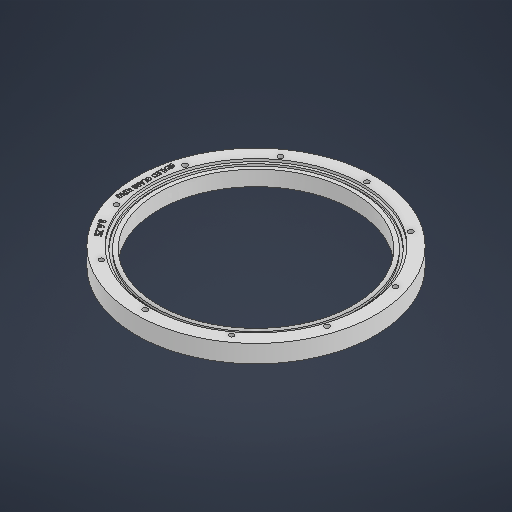
# Autodesk Inventor part: SealedGlassRing
Saved by Autodesk Inventor 2026.1 (Build 301233000, 233)
## iProperties
Created: 2025-06-19
Part Number: SealedGlassRing
Material: Generic
Document SubType Name: Modeling
Designer: mumin
Density: 1 g/cm^3
Appearance: Default
Author: mumin
Autodesk Inventor part; units mm, degrees
ref_plane "YZ Plane" through (0, 0, 0) normal (1, 0, 0) x (0, 1, 0)
ref_plane "XZ Plane" through (0, 0, 0) normal (0, 1, 0) x (-1, 0, 0)
ref_plane "XY Plane" through (0, 0, 0) normal (0, 0, 1) x (1, 0, 0)
sketch "Sketch1" plane through (0, 0, 0) normal (0, 1, 0) x (-1, 0, 0)
  circle A0 centre (0, 0) radius 110
  circle A1 centre (0, 0) radius 135
  dimension "d0" = 220
  dimension "d1" = 270
  constraints: 2 centre point, 2 coincident
  measures "d0" diameter of A0
  measures "d1" diameter of A1
extrude "Ring" add sketch "Sketch1" along normal blind 20
sketch "Sketch2" plane through (0, 20, 0) normal (0, 1, 0) x (1, 0, 0)
  circle A0 centre (0, 0) radius 120.5
  dimension "d4" = 241
  constraints: 1 centre point, 1 coincident
  measures "d4" diameter of A0
extrude "Glass Seat" cut sketch "Sketch2" against normal blind 2.95
sketch "Sketch3" plane through (0, 20, 0) normal (0, 1, 0) x (1, 0, 0)
  line L0 (0, 189) -> (0, -189) projected
  point P0 (0, 0)
  point P1 (0, 125)
  dimension "d14" = 125
  constraints: 1 point on line
  measures "d14" distance of point (0, 0) point (0, 125)
hole "Holes" at (0, 20, -125) direction (0, -1, 0) diameter 5.5 end through all
pattern_circular "Circular Pattern1" count 10 over 360 about axis through (0, -10, 0) along (0, 1, 0) of "Holes"
sketch "Sketch4" plane through (0, 20, 0) normal (0, 1, 0) x (1, 0, 0)
  line L0 (-123.4008, 33.078) -> (-123.4008, -40.8071) construction
  line L1 (-123.4008, -40.8071) -> (-126.5772, -40.8071) construction
  line L2 (-126.5772, -40.8071) -> (-126.5772, 33.078) construction
  line L3 (-126.5772, 33.078) -> (-123.4008, 33.078) construction
  spline S0 degree 2 poles (-128.5791, 31.1777) (-128.5791, 31.7207) (-128.3522, 32.4824) (-128.1901, 32.8187) knots 0 0 0 1 2 2 2
  line L4 (-128.1901, 32.8187) -> (-127.3554, 32.8187)
  line L5 (-127.3554, 32.8187) -> (-127.3554, 32.7701)
  spline S1 degree 2 poles (-127.3554, 32.7701) (-127.6634, 32.4419) (-128.0037, 31.6113) (-128.0037, 31.2263) knots 0 0 0 1 2 2 2
  spline S2 degree 2 poles (-128.0037, 31.2263) (-128.0037, 30.6753) (-127.5459, 30.1121) (-127.169, 30.1121) knots 0 0 0 1 2 2 2
  spline S3 degree 2 poles (-127.169, 30.1121) (-126.8692, 30.1121) (-126.4964, 30.4079) (-126.4032, 30.7279) knots 0 0 0 1 2 2 2
  spline S4 degree 2 poles (-126.4032, 30.7279) (-126.3384, 30.9589) (-126.2493, 31.3438) (-126.1763, 31.6315) knots 0 0 0 1 2 2 2
  spline S5 degree 2 poles (-126.1763, 31.6315) (-126.1074, 31.8908) (-125.9008, 32.3001) (-125.7347, 32.4581) knots 0 0 0 1 2 2 2
  spline S6 degree 2 poles (-125.7347, 32.4581) (-125.5685, 32.6121) (-125.1228, 32.7822) (-124.8311, 32.7822) knots 0 0 0 1 2 2 2
  spline S7 degree 2 poles (-124.8311, 32.7822) (-124.2233, 32.7822) (-123.4008, 31.8341) (-123.4008, 31.1007) knots 0 0 0 1 2 2 2
  spline S8 degree 2 poles (-123.4008, 31.1007) (-123.4008, 30.6793) (-123.5669, 29.9338) (-123.7249, 29.6137) knots 0 0 0 1 2 2 2
  line L6 (-123.7249, 29.6137) -> (-124.5191, 29.6137)
  line L7 (-124.5191, 29.6137) -> (-124.5191, 29.6623)
  spline S9 degree 2 poles (-124.5191, 29.6623) (-124.3003, 29.9014) (-123.9762, 30.6469) (-123.9762, 31.0561) knots 0 0 0 1 2 2 2
  spline S10 degree 2 poles (-123.9762, 31.0561) (-123.9762, 31.5181) (-124.4097, 32.0894) (-124.7622, 32.0894) knots 0 0 0 1 2 2 2
  spline S11 degree 2 poles (-124.7622, 32.0894) (-125.0783, 32.0894) (-125.4551, 31.7531) (-125.5402, 31.437) knots 0 0 0 1 2 2 2
  spline S12 degree 2 poles (-125.5402, 31.437) (-125.5969, 31.2263) (-125.7428, 30.6145) (-125.8036, 30.4119) knots 0 0 0 1 2 2 2
  spline S13 degree 2 poles (-125.8036, 30.4119) (-125.9616, 29.8973) (-126.5977, 29.4192) (-127.0637, 29.4192) knots 0 0 0 1 2 2 2
  spline S14 degree 2 poles (-127.0637, 29.4192) (-127.3595, 29.4192) (-127.9267, 29.6583) (-128.1253, 29.873) knots 0 0 0 1 2 2 2
  spline S15 degree 2 poles (-128.1253, 29.873) (-128.3441, 30.1121) (-128.5791, 30.7198) (-128.5791, 31.1777) knots 0 0 0 1 2 2 2
  line L8 (-128.4899, 28.7425) -> (-123.4899, 28.7425)
  line L9 (-123.4899, 28.7425) -> (-123.4899, 25.6145)
  line L10 (-123.4899, 25.6145) -> (-124.0815, 25.6145)
  line L11 (-124.0815, 25.6145) -> (-124.0815, 28.078)
  line L12 (-124.0815, 28.078) -> (-125.451, 28.078)
  line L13 (-125.451, 28.078) -> (-125.451, 25.7806)
  line L14 (-125.451, 25.7806) -> (-126.0426, 25.7806)
  line L15 (-126.0426, 25.7806) -> (-126.0426, 28.078)
  line L16 (-126.0426, 28.078) -> (-127.8984, 28.078)
  line L17 (-127.8984, 28.078) -> (-127.8984, 25.6145)
  line L18 (-127.8984, 25.6145) -> (-128.4899, 25.6145)
  line L19 (-128.4899, 25.6145) -> (-128.4899, 28.7425)
  line L20 (-128.4899, 25.4241) -> (-123.4899, 23.7385)
  line L21 (-123.4899, 23.7385) -> (-123.4899, 22.92)
  line L22 (-123.4899, 22.92) -> (-128.4899, 21.2344)
  line L23 (-128.4899, 21.2344) -> (-128.4899, 21.9354)
  line L24 (-128.4899, 21.9354) -> (-127.092, 22.3892)
  line L25 (-127.092, 22.3892) -> (-127.092, 24.2976)
  line L26 (-127.092, 24.2976) -> (-128.4899, 24.7514)
  line L27 (-128.4899, 24.7514) -> (-128.4899, 25.4241)
  line L28 (-126.5248, 22.5715) -> (-124.1707, 23.3455)
  line L29 (-124.1707, 23.3455) -> (-126.5248, 24.1153)
  line L30 (-126.5248, 24.1153) -> (-126.5248, 22.5715)
  line L31 (-128.4899, 17.8633) -> (-128.4899, 20.7604)
  line L32 (-128.4899, 20.7604) -> (-123.4899, 20.7604)
  line L33 (-123.4899, 20.7604) -> (-123.4899, 20.0959)
  line L34 (-123.4899, 20.0959) -> (-127.8984, 20.0959)
  line L35 (-127.8984, 20.0959) -> (-127.8984, 17.8633)
  line L36 (-127.8984, 17.8633) -> (-128.4899, 17.8633)
  line L37 (-128.4899, 17.3406) -> (-123.4899, 17.3406)
  line L38 (-123.4899, 17.3406) -> (-123.4899, 14.2126)
  line L39 (-123.4899, 14.2126) -> (-124.0815, 14.2126)
  line L40 (-124.0815, 14.2126) -> (-124.0815, 16.6761)
  line L41 (-124.0815, 16.6761) -> (-125.451, 16.6761)
  line L42 (-125.451, 16.6761) -> (-125.451, 14.3787)
  line L43 (-125.451, 14.3787) -> (-126.0426, 14.3787)
  line L44 (-126.0426, 14.3787) -> (-126.0426, 16.6761)
  line L45 (-126.0426, 16.6761) -> (-127.8984, 16.6761)
  line L46 (-127.8984, 16.6761) -> (-127.8984, 14.2126)
  line L47 (-127.8984, 14.2126) -> (-128.4899, 14.2126)
  line L48 (-128.4899, 14.2126) -> (-128.4899, 17.3406)
  spline S16 degree 2 poles (-125.994, 9.5408) (-126.6788, 9.5408) (-127.7809, 10.0959) (-128.0888, 10.5618) knots 0 0 0 1 2 2 2
  spline S17 degree 2 poles (-128.0888, 10.5618) (-128.3279, 10.9427) (-128.4899, 11.7247) (-128.4899, 12.3325) knots 0 0 0 1 2 2 2
  line L49 (-128.4899, 12.3325) -> (-128.4899, 13.4832)
  line L50 (-128.4899, 13.4832) -> (-123.4899, 13.4832)
  line L51 (-123.4899, 13.4832) -> (-123.4899, 12.3446)
  spline S18 degree 2 poles (-123.4899, 12.3446) (-123.4899, 11.6396) (-123.7006, 10.8373) (-123.887, 10.5537) knots 0 0 0 1 2 2 2
  spline S19 degree 2 poles (-123.887, 10.5537) (-124.2071, 10.0715) (-125.2647, 9.5408) (-125.994, 9.5408) knots 0 0 0 1 2 2 2
  spline S20 degree 2 poles (-125.9859, 10.2336) (-125.4105, 10.2336) (-124.5961, 10.6145) (-124.3651, 10.9913) knots 0 0 0 1 2 2 2
  spline S21 degree 2 poles (-124.3651, 10.9913) (-124.2071, 11.2587) (-124.0653, 11.8625) (-124.0653, 12.3122) knots 0 0 0 1 2 2 2
  line L52 (-124.0653, 12.3122) -> (-124.0653, 12.8187)
  line L53 (-124.0653, 12.8187) -> (-127.9146, 12.8187)
  line L54 (-127.9146, 12.8187) -> (-127.9146, 12.3122)
  spline S22 degree 2 poles (-127.9146, 12.3122) (-127.9146, 11.8706) (-127.7728, 11.202) (-127.5823, 10.9305) knots 0 0 0 1 2 2 2
  spline S23 degree 2 poles (-127.5823, 10.9305) (-127.3473, 10.5821) (-126.5694, 10.2336) (-125.9859, 10.2336) knots 0 0 0 1 2 2 2
  spline S24 degree 2 poles (-128.5872, 4.5772) (-128.5872, 5.108) (-128.263, 5.9873) (-127.9348, 6.3033) knots 0 0 0 1 2 2 2
  spline S25 degree 2 poles (-127.9348, 6.3033) (-127.6026, 6.6194) (-126.622, 6.9557) (-125.9859, 6.9557) knots 0 0 0 1 2 2 2
  spline S26 degree 2 poles (-125.9859, 6.9557) (-125.3822, 6.9557) (-124.4259, 6.6153) (-124.0856, 6.2993) knots 0 0 0 1 2 2 2
  spline S27 degree 2 poles (-124.0856, 6.2993) (-123.7574, 5.9954) (-123.4008, 5.104) (-123.4008, 4.5732) knots 0 0 0 1 2 2 2
  spline S28 degree 2 poles (-123.4008, 4.5732) (-123.4008, 4.3179) (-123.4737, 3.856) (-123.5386, 3.6453) knots 0 0 0 1 2 2 2
  spline S29 degree 2 poles (-123.5386, 3.6453) (-123.5872, 3.4751) (-123.7655, 3.0618) (-123.8303, 2.9362) knots 0 0 0 1 2 2 2
  line L55 (-123.8303, 2.9362) -> (-124.6326, 2.9362)
  line L56 (-124.6326, 2.9362) -> (-124.6326, 2.9929)
  spline S30 degree 2 poles (-124.6326, 2.9929) (-124.5232, 3.1185) (-124.3246, 3.3819) (-124.2112, 3.625) knots 0 0 0 1 2 2 2
  spline S31 degree 2 poles (-124.2112, 3.625) (-124.1099, 3.8276) (-123.9762, 4.3503) (-123.9762, 4.6502) knots 0 0 0 1 2 2 2
  spline S32 degree 2 poles (-123.9762, 4.6502) (-123.9762, 5.3714) (-125.0621, 6.2628) (-125.9656, 6.2628) knots 0 0 0 1 2 2 2
  spline S33 degree 2 poles (-125.9656, 6.2628) (-126.4681, 6.2628) (-127.2217, 6.0278) (-127.481, 5.8049) knots 0 0 0 1 2 2 2
  spline S34 degree 2 poles (-127.481, 5.8049) (-127.7403, 5.5902) (-128.0118, 4.9824) (-128.0118, 4.6015) knots 0 0 0 1 2 2 2
  spline S35 degree 2 poles (-128.0118, 4.6015) (-128.0118, 4.322) (-127.9308, 3.7628) (-127.8497, 3.5724) knots 0 0 0 1 2 2 2
  line L57 (-127.8497, 3.5724) -> (-126.5572, 3.5724)
  line L58 (-126.5572, 3.5724) -> (-126.5572, 4.7312)
  line L59 (-126.5572, 4.7312) -> (-125.9737, 4.7312)
  line L60 (-125.9737, 4.7312) -> (-125.9737, 2.916)
  line L61 (-125.9737, 2.916) -> (-128.1577, 2.916)
  spline S36 degree 2 poles (-128.1577, 2.916) (-128.2144, 3.0416) (-128.3886, 3.4711) (-128.4413, 3.6534) knots 0 0 0 1 2 2 2
  spline S37 degree 2 poles (-128.4413, 3.6534) (-128.5142, 3.9006) (-128.5872, 4.2976) (-128.5872, 4.5772) knots 0 0 0 1 2 2 2
  line L62 (-128.4899, -0.8158) -> (-128.4899, 2.0813)
  line L63 (-128.4899, 2.0813) -> (-123.4899, 2.0813)
  line L64 (-123.4899, 2.0813) -> (-123.4899, 1.4168)
  line L65 (-123.4899, 1.4168) -> (-127.8984, 1.4168)
  line L66 (-127.8984, 1.4168) -> (-127.8984, -0.8158)
  line L67 (-127.8984, -0.8158) -> (-128.4899, -0.8158)
  line L68 (-128.4899, -0.7996) -> (-123.4899, -2.4852)
  line L69 (-123.4899, -2.4852) -> (-123.4899, -3.3037)
  line L70 (-123.4899, -3.3037) -> (-128.4899, -4.9892)
  line L71 (-128.4899, -4.9892) -> (-128.4899, -4.2883)
  line L72 (-128.4899, -4.2883) -> (-127.092, -3.8345)
  line L73 (-127.092, -3.8345) -> (-127.092, -1.926)
  line L74 (-127.092, -1.926) -> (-128.4899, -1.4722)
  line L75 (-128.4899, -1.4722) -> (-128.4899, -0.7996)
  line L76 (-126.5248, -3.6521) -> (-124.1707, -2.8782)
  line L77 (-124.1707, -2.8782) -> (-126.5248, -2.1084)
  line L78 (-126.5248, -2.1084) -> (-126.5248, -3.6521)
  spline S38 degree 2 poles (-128.5791, -6.8571) (-128.5791, -6.3142) (-128.3522, -5.5524) (-128.1901, -5.2161) knots 0 0 0 1 2 2 2
  line L79 (-128.1901, -5.2161) -> (-127.3554, -5.2161)
  line L80 (-127.3554, -5.2161) -> (-127.3554, -5.2648)
  spline S39 degree 2 poles (-127.3554, -5.2648) (-127.6634, -5.593) (-128.0037, -6.4236) (-128.0037, -6.8085) knots 0 0 0 1 2 2 2
  spline S40 degree 2 poles (-128.0037, -6.8085) (-128.0037, -7.3596) (-127.5459, -7.9228) (-127.169, -7.9228) knots 0 0 0 1 2 2 2
  spline S41 degree 2 poles (-127.169, -7.9228) (-126.8692, -7.9228) (-126.4964, -7.627) (-126.4032, -7.3069) knots 0 0 0 1 2 2 2
  spline S42 degree 2 poles (-126.4032, -7.3069) (-126.3384, -7.0759) (-126.2493, -6.691) (-126.1763, -6.4033) knots 0 0 0 1 2 2 2
  spline S43 degree 2 poles (-126.1763, -6.4033) (-126.1074, -6.144) (-125.9008, -5.7348) (-125.7347, -5.5768) knots 0 0 0 1 2 2 2
  spline S44 degree 2 poles (-125.7347, -5.5768) (-125.5685, -5.4228) (-125.1228, -5.2526) (-124.8311, -5.2526) knots 0 0 0 1 2 2 2
  spline S45 degree 2 poles (-124.8311, -5.2526) (-124.2233, -5.2526) (-123.4008, -6.2007) (-123.4008, -6.9341) knots 0 0 0 1 2 2 2
  spline S46 degree 2 poles (-123.4008, -6.9341) (-123.4008, -7.3555) (-123.5669, -8.1011) (-123.7249, -8.4212) knots 0 0 0 1 2 2 2
  line L81 (-123.7249, -8.4212) -> (-124.5191, -8.4212)
  line L82 (-124.5191, -8.4212) -> (-124.5191, -8.3725)
  spline S47 degree 2 poles (-124.5191, -8.3725) (-124.3003, -8.1335) (-123.9762, -7.3879) (-123.9762, -6.9787) knots 0 0 0 1 2 2 2
  spline S48 degree 2 poles (-123.9762, -6.9787) (-123.9762, -6.5168) (-124.4097, -5.9455) (-124.7622, -5.9455) knots 0 0 0 1 2 2 2
  spline S49 degree 2 poles (-124.7622, -5.9455) (-125.0783, -5.9455) (-125.4551, -6.2818) (-125.5402, -6.5978) knots 0 0 0 1 2 2 2
  spline S50 degree 2 poles (-125.5402, -6.5978) (-125.5969, -6.8085) (-125.7428, -7.4203) (-125.8036, -7.6229) knots 0 0 0 1 2 2 2
  spline S51 degree 2 poles (-125.8036, -7.6229) (-125.9616, -8.1375) (-126.5977, -8.6156) (-127.0637, -8.6156) knots 0 0 0 1 2 2 2
  spline S52 degree 2 poles (-127.0637, -8.6156) (-127.3595, -8.6156) (-127.9267, -8.3766) (-128.1253, -8.1618) knots 0 0 0 1 2 2 2
  spline S53 degree 2 poles (-128.1253, -8.1618) (-128.3441, -7.9228) (-128.5791, -7.315) (-128.5791, -6.8571) knots 0 0 0 1 2 2 2
  spline S54 degree 2 poles (-128.5791, -10.6862) (-128.5791, -10.1432) (-128.3522, -9.3815) (-128.1901, -9.0451) knots 0 0 0 1 2 2 2
  line L83 (-128.1901, -9.0451) -> (-127.3554, -9.0451)
  line L84 (-127.3554, -9.0451) -> (-127.3554, -9.0938)
  spline S55 degree 2 poles (-127.3554, -9.0938) (-127.6634, -9.422) (-128.0037, -10.2526) (-128.0037, -10.6375) knots 0 0 0 1 2 2 2
  spline S56 degree 2 poles (-128.0037, -10.6375) (-128.0037, -11.1886) (-127.5459, -11.7518) (-127.169, -11.7518) knots 0 0 0 1 2 2 2
  spline S57 degree 2 poles (-127.169, -11.7518) (-126.8692, -11.7518) (-126.4964, -11.456) (-126.4032, -11.1359) knots 0 0 0 1 2 2 2
  spline S58 degree 2 poles (-126.4032, -11.1359) (-126.3384, -10.905) (-126.2493, -10.52) (-126.1763, -10.2323) knots 0 0 0 1 2 2 2
  spline S59 degree 2 poles (-126.1763, -10.2323) (-126.1074, -9.973) (-125.9008, -9.5638) (-125.7347, -9.4058) knots 0 0 0 1 2 2 2
  spline S60 degree 2 poles (-125.7347, -9.4058) (-125.5685, -9.2518) (-125.1228, -9.0816) (-124.8311, -9.0816) knots 0 0 0 1 2 2 2
  spline S61 degree 2 poles (-124.8311, -9.0816) (-124.2233, -9.0816) (-123.4008, -10.0298) (-123.4008, -10.7631) knots 0 0 0 1 2 2 2
  spline S62 degree 2 poles (-123.4008, -10.7631) (-123.4008, -11.1845) (-123.5669, -11.9301) (-123.7249, -12.2502) knots 0 0 0 1 2 2 2
  line L85 (-123.7249, -12.2502) -> (-124.5191, -12.2502)
  line L86 (-124.5191, -12.2502) -> (-124.5191, -12.2015)
  spline S63 degree 2 poles (-124.5191, -12.2015) (-124.3003, -11.9625) (-123.9762, -11.2169) (-123.9762, -10.8077) knots 0 0 0 1 2 2 2
  spline S64 degree 2 poles (-123.9762, -10.8077) (-123.9762, -10.3458) (-124.4097, -9.7745) (-124.7622, -9.7745) knots 0 0 0 1 2 2 2
  spline S65 degree 2 poles (-124.7622, -9.7745) (-125.0783, -9.7745) (-125.4551, -10.1108) (-125.5402, -10.4268) knots 0 0 0 1 2 2 2
  spline S66 degree 2 poles (-125.5402, -10.4268) (-125.5969, -10.6375) (-125.7428, -11.2494) (-125.8036, -11.452) knots 0 0 0 1 2 2 2
  spline S67 degree 2 poles (-125.8036, -11.452) (-125.9616, -11.9665) (-126.5977, -12.4447) (-127.0637, -12.4447) knots 0 0 0 1 2 2 2
  spline S68 degree 2 poles (-127.0637, -12.4447) (-127.3595, -12.4447) (-127.9267, -12.2056) (-128.1253, -11.9909) knots 0 0 0 1 2 2 2
  spline S69 degree 2 poles (-128.1253, -11.9909) (-128.3441, -11.7518) (-128.5791, -11.144) (-128.5791, -10.6862) knots 0 0 0 1 2 2 2
  line L87 (-128.4899, -19.1383) -> (-128.4899, -18.2753)
  line L88 (-128.4899, -18.2753) -> (-126.5005, -16.6951)
  line L89 (-126.5005, -16.6951) -> (-126.5005, -15.9333)
  line L90 (-126.5005, -15.9333) -> (-128.4899, -15.9333)
  line L91 (-128.4899, -15.9333) -> (-128.4899, -15.2688)
  line L92 (-128.4899, -15.2688) -> (-123.4899, -15.2688)
  line L93 (-123.4899, -15.2688) -> (-123.4899, -16.5573)
  spline S70 degree 2 poles (-123.4899, -16.5573) (-123.4899, -16.9868) (-123.5831, -17.5662) (-123.7533, -17.8296) knots 0 0 0 1 2 2 2
  spline S71 degree 2 poles (-123.7533, -17.8296) (-123.9235, -18.093) (-124.4543, -18.3968) (-124.8473, -18.3968) knots 0 0 0 1 2 2 2
  spline S72 degree 2 poles (-124.8473, -18.3968) (-125.3943, -18.3968) (-126.1358, -17.8377) (-126.3141, -17.3596) knots 0 0 0 1 2 2 2
  line L94 (-126.3141, -17.3596) -> (-128.4899, -19.1383)
  spline S73 degree 2 poles (-124.9, -17.704) (-124.6812, -17.704) (-124.3449, -17.55) (-124.2355, -17.3879) knots 0 0 0 1 2 2 2
  spline S74 degree 2 poles (-124.2355, -17.3879) (-124.1423, -17.2461) (-124.0653, -16.8693) (-124.0653, -16.5938) knots 0 0 0 1 2 2 2
  line L95 (-124.0653, -16.5938) -> (-124.0653, -15.9333)
  line L96 (-124.0653, -15.9333) -> (-125.9454, -15.9333)
  line L97 (-125.9454, -15.9333) -> (-125.9454, -16.5168)
  spline S75 degree 2 poles (-125.9454, -16.5168) (-125.9454, -16.8045) (-125.8441, -17.2623) (-125.686, -17.4203) knots 0 0 0 1 2 2 2
  spline S76 degree 2 poles (-125.686, -17.4203) (-125.5483, -17.5662) (-125.1593, -17.704) (-124.9, -17.704) knots 0 0 0 1 2 2 2
  line L98 (-128.4899, -21.2777) -> (-128.4899, -19.3409)
  line L99 (-128.4899, -19.3409) -> (-127.9794, -19.3409)
  line L100 (-127.9794, -19.3409) -> (-127.9794, -19.9771)
  line L101 (-127.9794, -19.9771) -> (-124.0005, -19.9771)
  line L102 (-124.0005, -19.9771) -> (-124.0005, -19.3409)
  line L103 (-124.0005, -19.3409) -> (-123.4899, -19.3409)
  line L104 (-123.4899, -19.3409) -> (-123.4899, -21.2777)
  line L105 (-123.4899, -21.2777) -> (-124.0005, -21.2777)
  line L106 (-124.0005, -21.2777) -> (-124.0005, -20.6416)
  line L107 (-124.0005, -20.6416) -> (-127.9794, -20.6416)
  line L108 (-127.9794, -20.6416) -> (-127.9794, -21.2777)
  line L109 (-127.9794, -21.2777) -> (-128.4899, -21.2777)
  line L110 (-128.4899, -25.678) -> (-128.4899, -24.9325)
  line L111 (-128.4899, -24.9325) -> (-124.1788, -22.7202)
  line L112 (-124.1788, -22.7202) -> (-128.4899, -22.7202)
  line L113 (-128.4899, -22.7202) -> (-128.4899, -22.1003)
  line L114 (-128.4899, -22.1003) -> (-123.4899, -22.1003)
  line L115 (-123.4899, -22.1003) -> (-123.4899, -23.0443)
  line L116 (-123.4899, -23.0443) -> (-127.4486, -25.0581)
  line L117 (-127.4486, -25.0581) -> (-123.4899, -25.0581)
  line L118 (-123.4899, -25.0581) -> (-123.4899, -25.678)
  line L119 (-123.4899, -25.678) -> (-128.4899, -25.678)
  spline S77 degree 2 poles (-128.5872, -28.7858) (-128.5872, -28.255) (-128.263, -27.3758) (-127.9348, -27.0597) knots 0 0 0 1 2 2 2
  spline S78 degree 2 poles (-127.9348, -27.0597) (-127.6026, -26.7437) (-126.622, -26.4074) (-125.9859, -26.4074) knots 0 0 0 1 2 2 2
  spline S79 degree 2 poles (-125.9859, -26.4074) (-125.3822, -26.4074) (-124.4259, -26.7477) (-124.0856, -27.0638) knots 0 0 0 1 2 2 2
  spline S80 degree 2 poles (-124.0856, -27.0638) (-123.7574, -27.3677) (-123.4008, -28.2591) (-123.4008, -28.7899) knots 0 0 0 1 2 2 2
  spline S81 degree 2 poles (-123.4008, -28.7899) (-123.4008, -29.0451) (-123.4737, -29.5071) (-123.5386, -29.7178) knots 0 0 0 1 2 2 2
  spline S82 degree 2 poles (-123.5386, -29.7178) (-123.5872, -29.8879) (-123.7655, -30.3012) (-123.8303, -30.4268) knots 0 0 0 1 2 2 2
  line L120 (-123.8303, -30.4268) -> (-124.6326, -30.4268)
  line L121 (-124.6326, -30.4268) -> (-124.6326, -30.3701)
  spline S83 degree 2 poles (-124.6326, -30.3701) (-124.5232, -30.2445) (-124.3246, -29.9811) (-124.2112, -29.738) knots 0 0 0 1 2 2 2
  spline S84 degree 2 poles (-124.2112, -29.738) (-124.1099, -29.5354) (-123.9762, -29.0127) (-123.9762, -28.7129) knots 0 0 0 1 2 2 2
  spline S85 degree 2 poles (-123.9762, -28.7129) (-123.9762, -27.9917) (-125.0621, -27.1003) (-125.9656, -27.1003) knots 0 0 0 1 2 2 2
  spline S86 degree 2 poles (-125.9656, -27.1003) (-126.4681, -27.1003) (-127.2217, -27.3353) (-127.481, -27.5581) knots 0 0 0 1 2 2 2
  spline S87 degree 2 poles (-127.481, -27.5581) (-127.7403, -27.7729) (-128.0118, -28.3806) (-128.0118, -28.7615) knots 0 0 0 1 2 2 2
  spline S88 degree 2 poles (-128.0118, -28.7615) (-128.0118, -29.0411) (-127.9308, -29.6003) (-127.8497, -29.7907) knots 0 0 0 1 2 2 2
  line L122 (-127.8497, -29.7907) -> (-126.5572, -29.7907)
  line L123 (-126.5572, -29.7907) -> (-126.5572, -28.6319)
  line L124 (-126.5572, -28.6319) -> (-125.9737, -28.6319)
  line L125 (-125.9737, -28.6319) -> (-125.9737, -30.4471)
  line L126 (-125.9737, -30.4471) -> (-128.1577, -30.4471)
  spline S89 degree 2 poles (-128.1577, -30.4471) (-128.2144, -30.3215) (-128.3886, -29.892) (-128.4413, -29.7097) knots 0 0 0 1 2 2 2
  spline S90 degree 2 poles (-128.4413, -29.7097) (-128.5142, -29.4625) (-128.5872, -29.0654) (-128.5872, -28.7858) knots 0 0 0 1 2 2 2
  point P0 (0, 0)
  constraints: 2 other
emboss "Emboss1" sketch "Sketch4" operation cut depth 1 direction (0, -1, 0)
sketch "Sketch5" plane through (0, 17.05, 0) normal (0, 1, 0) x (1, 0, 0)
  circle A0 centre (0, 0) radius 120.5 projected
  circle A1 centre (0, 0) radius 117.5
  circle A2 centre (0, 0) radius 114.5
  dimension "d25" = 3
  dimension "d26" = 3
  constraints: 2 centre point
  measures "d25" radial gap between concentric circles of A0 A1
  measures "d26" radial gap between concentric circles of A1 A2
extrude "Seal Groove" cut sketch "Sketch5" against normal blind 2.5 contours A1
sketch "Sketch6" plane through (0, 20, 0) normal (0, 1, 0) x (1, 0, 0)
  line L0 (-109.3924, -58.9981) -> (-82.8013, -97.4436) construction
  line L1 (-82.8013, -97.4436) -> (-85.9073, -99.5919) construction
  line L2 (-85.9073, -99.5919) -> (-112.4984, -61.1464) construction
  line L3 (-112.4984, -61.1464) -> (-109.3924, -58.9981) construction
  spline S0 degree 2 poles (-113.2704, -64.4176) (-113.5249, -64.0497) (-113.7226, -63.2937) (-113.6652, -62.9407) knots 0 0 0 1 2 2 2
  spline S1 degree 2 poles (-113.6652, -62.9407) (-113.6091, -62.5945) (-113.2146, -62.0024) (-112.9067, -61.7894) knots 0 0 0 1 2 2 2
  spline S2 degree 2 poles (-112.9067, -61.7894) (-112.5068, -61.5128) (-111.539, -61.476) (-111.057, -61.7456) knots 0 0 0 1 2 2 2
  line L4 (-111.057, -61.7456) -> (-111.037, -61.7318)
  spline S3 degree 2 poles (-111.037, -61.7318) (-111.0767, -61.2213) (-110.8163, -60.5209) (-110.4404, -60.2609) knots 0 0 0 1 2 2 2
  spline S4 degree 2 poles (-110.4404, -60.2609) (-109.8845, -59.8765) (-108.5599, -60.2018) (-108.1118, -60.8496) knots 0 0 0 1 2 2 2
  spline S5 degree 2 poles (-108.1118, -60.8496) (-107.6471, -61.5214) (-107.7895, -62.82) (-108.3413, -63.2017) knots 0 0 0 1 2 2 2
  spline S6 degree 2 poles (-108.3413, -63.2017) (-108.6732, -63.4312) (-109.5893, -63.4914) (-110.025, -63.2547) knots 0 0 0 1 2 2 2
  line L5 (-110.025, -63.2547) -> (-110.045, -63.2686)
  spline S7 degree 2 poles (-110.045, -63.2686) (-109.9462, -63.8388) (-110.215, -64.6809) (-110.6709, -64.9962) knots 0 0 0 1 2 2 2
  spline S8 degree 2 poles (-110.6709, -64.9962) (-111.3027, -65.4332) (-112.7947, -65.1054) (-113.2704, -64.4176) knots 0 0 0 1 2 2 2
  spline S9 degree 2 poles (-111.2051, -64.3607) (-110.9012, -64.1505) (-110.7072, -63.6616) (-110.7584, -63.1945) knots 0 0 0 1 2 2 2
  spline S10 degree 2 poles (-110.7584, -63.1945) (-110.7718, -63.0382) (-110.8839, -62.56) (-110.9511, -62.2577) knots 0 0 0 1 2 2 2
  spline S11 degree 2 poles (-110.9511, -62.2577) (-111.3191, -62.1102) (-112.0569, -62.1889) (-112.3968, -62.424) knots 0 0 0 1 2 2 2
  spline S12 degree 2 poles (-112.3968, -62.424) (-112.8447, -62.7338) (-113.0551, -63.6775) (-112.773, -64.0854) knots 0 0 0 1 2 2 2
  spline S13 degree 2 poles (-112.773, -64.0854) (-112.4853, -64.5013) (-111.637, -64.6594) (-111.2051, -64.3607) knots 0 0 0 1 2 2 2
  spline S14 degree 2 poles (-108.7974, -62.5594) (-108.4655, -62.3298) (-108.3286, -61.5789) (-108.6024, -61.183) knots 0 0 0 1 2 2 2
  spline S15 degree 2 poles (-108.6024, -61.183) (-108.8514, -60.8231) (-109.5653, -60.6371) (-109.9052, -60.8722) knots 0 0 0 1 2 2 2
  spline S16 degree 2 poles (-109.9052, -60.8722) (-110.1492, -61.0409) (-110.3259, -61.5119) (-110.2987, -61.8419) knots 0 0 0 1 2 2 2
  spline S17 degree 2 poles (-110.2987, -61.8419) (-110.2855, -61.9806) (-110.1883, -62.54) (-110.1253, -62.7507) knots 0 0 0 1 2 2 2
  spline S18 degree 2 poles (-110.1253, -62.7507) (-109.7062, -62.8865) (-109.0973, -62.7668) (-108.7974, -62.5594) knots 0 0 0 1 2 2 2
  line L6 (-110.8959, -67.6112) -> (-111.4436, -66.8195)
  line L7 (-111.4436, -66.8195) -> (-110.4998, -66.1667)
  line L8 (-110.4998, -66.1667) -> (-109.9522, -66.9585)
  line L9 (-109.9522, -66.9585) -> (-110.8959, -67.6112)
  spline S19 degree 2 poles (-106.4503, -70.6198) (-106.8302, -70.8825) (-107.6483, -71.0759) (-108.0108, -71.0133) knots 0 0 0 1 2 2 2
  spline S20 degree 2 poles (-108.0108, -71.0133) (-108.3908, -70.951) (-109.0085, -70.5624) (-109.238, -70.2305) knots 0 0 0 1 2 2 2
  spline S21 degree 2 poles (-109.238, -70.2305) (-109.4676, -69.8985) (-109.6226, -69.1958) (-109.5425, -68.833) knots 0 0 0 1 2 2 2
  spline S22 degree 2 poles (-109.5425, -68.833) (-109.4516, -68.3917) (-108.751, -67.4815) (-108.0951, -67.0279) knots 0 0 0 1 2 2 2
  spline S23 degree 2 poles (-108.0951, -67.0279) (-107.4513, -66.5826) (-106.2331, -66.1301) (-105.6583, -66.1405) knots 0 0 0 1 2 2 2
  spline S24 degree 2 poles (-105.6583, -66.1405) (-105.0971, -66.1485) (-104.0909, -66.7058) (-103.7064, -67.2617) knots 0 0 0 1 2 2 2
  spline S25 degree 2 poles (-103.7064, -67.2617) (-103.593, -67.4256) (-103.4258, -67.7357) (-103.3872, -67.8685) knots 0 0 0 1 2 2 2
  line L10 (-103.3872, -67.8685) -> (-104.023, -68.3083)
  line L11 (-104.023, -68.3083) -> (-104.0423, -68.2803)
  spline S26 degree 2 poles (-104.0423, -68.2803) (-104.058, -68.1552) (-104.2063, -67.7612) (-104.3391, -67.5692) knots 0 0 0 1 2 2 2
  spline S27 degree 2 poles (-104.3391, -67.5692) (-104.765, -66.9534) (-106.1196, -66.7729) (-106.9851, -67.2652) knots 0 0 0 1 2 2 2
  spline S28 degree 2 poles (-106.9851, -67.2652) (-106.658, -67.3877) (-106.1351, -67.7591) (-105.9304, -68.055) knots 0 0 0 1 2 2 2
  spline S29 degree 2 poles (-105.9304, -68.055) (-105.7312, -68.3429) (-105.5485, -68.855) (-105.5613, -69.2127) knots 0 0 0 1 2 2 2
  spline S30 degree 2 poles (-105.5613, -69.2127) (-105.5771, -69.6256) (-106.0264, -70.3266) (-106.4503, -70.6198) knots 0 0 0 1 2 2 2
  spline S31 degree 2 poles (-106.9429, -69.9673) (-106.639, -69.7571) (-106.3378, -69.3123) (-106.3155, -69.0367) knots 0 0 0 1 2 2 2
  spline S32 degree 2 poles (-106.3155, -69.0367) (-106.3028, -68.8329) (-106.4616, -68.4579) (-106.5806, -68.286) knots 0 0 0 1 2 2 2
  spline S33 degree 2 poles (-106.5806, -68.286) (-106.741, -68.054) (-107.1824, -67.715) (-107.461, -67.5943) knots 0 0 0 1 2 2 2
  spline S34 degree 2 poles (-107.461, -67.5943) (-107.5357, -67.6401) (-107.6772, -67.7261) (-107.7812, -67.798) knots 0 0 0 1 2 2 2
  spline S35 degree 2 poles (-107.7812, -67.798) (-108.2931, -68.1521) (-108.7826, -68.7863) (-108.8414, -69.0516) knots 0 0 0 1 2 2 2
  spline S36 degree 2 poles (-108.8414, -69.0516) (-108.9006, -69.2994) (-108.8144, -69.6891) (-108.6954, -69.8611) knots 0 0 0 1 2 2 2
  spline S37 degree 2 poles (-108.6954, -69.8611) (-108.4188, -70.261) (-107.5108, -70.3601) (-106.9429, -69.9673) knots 0 0 0 1 2 2 2
  line L12 (-106.9131, -73.3697) -> (-107.4607, -72.5779)
  line L13 (-107.4607, -72.5779) -> (-106.517, -71.9251)
  line L14 (-106.517, -71.9251) -> (-105.9693, -72.7169)
  line L15 (-105.9693, -72.7169) -> (-106.9131, -73.3697)
  line L16 (-104.1195, -77.4086) -> (-106.2244, -74.3654)
  line L17 (-106.2244, -74.3654) -> (-105.5246, -73.8814)
  spline S38 degree 2 poles (-105.5246, -73.8814) (-104.9898, -73.9963) (-104.0142, -74.1846) (-103.5127, -74.2516) knots 0 0 0 1 2 2 2
  spline S39 degree 2 poles (-103.5127, -74.2516) (-102.5028, -74.3867) (-101.4742, -74.2841) (-101.0783, -74.0103) knots 0 0 0 1 2 2 2
  spline S40 degree 2 poles (-101.0783, -74.0103) (-100.8703, -73.8665) (-100.6469, -73.5228) (-100.6271, -73.3377) knots 0 0 0 1 2 2 2
  spline S41 degree 2 poles (-100.6271, -73.3377) (-100.6074, -73.1526) (-100.7176, -72.7795) (-100.8448, -72.5955) knots 0 0 0 1 2 2 2
  spline S42 degree 2 poles (-100.8448, -72.5955) (-100.9665, -72.4196) (-101.3035, -72.1205) (-101.4848, -72.0036) knots 0 0 0 1 2 2 2
  spline S43 degree 2 poles (-101.4848, -72.0036) (-101.6376, -71.9024) (-101.9774, -71.7531) (-102.0887, -71.7118) knots 0 0 0 1 2 2 2
  line L18 (-102.0887, -71.7118) -> (-102.1136, -71.6758)
  line L19 (-102.1136, -71.6758) -> (-101.4098, -71.189)
  spline S44 degree 2 poles (-101.4098, -71.189) (-101.1687, -71.3238) (-100.4666, -71.9201) (-100.2398, -72.248) knots 0 0 0 1 2 2 2
  spline S45 degree 2 poles (-100.2398, -72.248) (-99.7613, -72.9398) (-99.9538, -74.2258) (-100.5776, -74.6572) knots 0 0 0 1 2 2 2
  spline S46 degree 2 poles (-100.5776, -74.6572) (-100.8695, -74.8592) (-101.4514, -75.0606) (-101.7423, -75.0845) knots 0 0 0 1 2 2 2
  spline S47 degree 2 poles (-101.7423, -75.0845) (-102.0413, -75.1139) (-102.7058, -75.0592) (-103.0425, -75.0083) knots 0 0 0 1 2 2 2
  spline S48 degree 2 poles (-103.0425, -75.0083) (-103.5981, -74.9315) (-104.8542, -74.671) (-105.2238, -74.5897) knots 0 0 0 1 2 2 2
  line L20 (-105.2238, -74.5897) -> (-103.5477, -77.013)
  line L21 (-103.5477, -77.013) -> (-104.1195, -77.4086)
  spline S49 degree 2 poles (-100.0267, -79.9753) (-100.3826, -80.2215) (-101.1481, -80.414) (-101.5159, -80.3609) knots 0 0 0 1 2 2 2
  spline S50 degree 2 poles (-101.5159, -80.3609) (-101.8836, -80.3079) (-102.5723, -79.8678) (-102.8378, -79.4839) knots 0 0 0 1 2 2 2
  spline S51 degree 2 poles (-102.8378, -79.4839) (-103.0812, -79.132) (-103.401, -78.3363) (-103.4513, -77.9987) knots 0 0 0 1 2 2 2
  line L22 (-103.4513, -77.9987) -> (-102.7514, -77.5146)
  line L23 (-102.7514, -77.5146) -> (-102.7183, -77.5626)
  spline S52 degree 2 poles (-102.7183, -77.5626) (-102.7217, -77.6773) (-102.6693, -78.0608) (-102.6143, -78.277) knots 0 0 0 1 2 2 2
  spline S53 degree 2 poles (-102.6143, -78.277) (-102.5468, -78.52) (-102.3987, -78.8965) (-102.2577, -79.1004) knots 0 0 0 1 2 2 2
  spline S54 degree 2 poles (-102.2577, -79.1004) (-102.1194, -79.3003) (-101.7154, -79.5767) (-101.4654, -79.6048) knots 0 0 0 1 2 2 2
  spline S55 degree 2 poles (-101.4654, -79.6048) (-101.2317, -79.6264) (-100.7513, -79.4833) (-100.4874, -79.3008) knots 0 0 0 1 2 2 2
  spline S56 degree 2 poles (-100.4874, -79.3008) (-100.2235, -79.1182) (-99.9871, -78.7419) (-99.9692, -78.5285) knots 0 0 0 1 2 2 2
  spline S57 degree 2 poles (-99.9692, -78.5285) (-99.942, -78.3028) (-100.1257, -77.815) (-100.3, -77.5631) knots 0 0 0 1 2 2 2
  spline S58 degree 2 poles (-100.3, -77.5631) (-100.488, -77.2911) (-100.9454, -76.8094) (-101.0948, -76.6703) knots 0 0 0 1 2 2 2
  line L24 (-101.0948, -76.6703) -> (-98.5515, -74.9112)
  line L25 (-98.5515, -74.9112) -> (-96.679, -77.6185)
  line L26 (-96.679, -77.6185) -> (-97.2588, -78.0195)
  line L27 (-97.2588, -78.0195) -> (-98.6916, -75.9481)
  line L28 (-98.6916, -75.9481) -> (-100.0072, -76.8581)
  spline S59 degree 2 poles (-100.0072, -76.8581) (-99.9082, -76.967) (-99.7358, -77.1906) (-99.6694, -77.2866) knots 0 0 0 1 2 2 2
  spline S60 degree 2 poles (-99.6694, -77.2866) (-99.4067, -77.6665) (-99.1683, -78.2761) (-99.1863, -78.6432) knots 0 0 0 1 2 2 2
  spline S61 degree 2 poles (-99.1863, -78.6432) (-99.2015, -79.0144) (-99.5788, -79.6656) (-100.0267, -79.9753) knots 0 0 0 1 2 2 2
  point P0 (0, 0)
  constraints: 2 other
emboss "Emboss2" sketch "Sketch6" operation cut depth 1 direction (0, -1, 0)
body "Solid1"
